# Autodesk Inventor part: Roller Chain
Saved by Autodesk Inventor 2016 (Build 200138000, 138)
## iProperties
Created: 2016-05-10
Part Number: Roller Chain
Material: Generic
Document SubType Name: Modeling
Designer: hesaon
Density: 1 g/cm^3
Appearance: Clear - Blue
CustomPartVersion: 1
Author: hesaon
Autodesk Inventor part; units mm, degrees
ref_plane "Work Plane2" through (-104.6542, 0, 0) normal (-1, 0, 0) x (0, 0, 1)
ref_plane "Work Plane3" through (200, 0, 0) normal (-0.9133742, 0.4071211, 0) x (0, 0, 1)
sketch "Path" plane through (0, 0, 0) normal (0, 0, 1) x (1, 0, 0)
  arc A0 (-103.7053, 31.9399) -> (-103.7053, -31.9399) centre (-104.6542, 0) ccw
  arc A1 (200.6803, -22.8963) -> (200.6803, 22.8963) centre (200, 0) ccw
  line L0 (200.6803, -22.8963) -> (-103.7053, -31.9399)
  line L1 (-103.7053, 31.9399) -> (200.6803, 22.8963)
  dimension "d31" = 8.26
  constraints: 4 end point, 4 point on circle, 2 centre point
ref_plane "Section Plane" through (-103.7053, -31.9399, 0) normal (0.9995589, 0.0296981, 0) x (0, 0, 1)
sketch "Section Sketch" plane through (-103.7053, -31.9399, 0) normal (0.9995589, 0.0296981, 0) x (0, 0, 1)
  line L0 (-6.75, -1.64) -> (6.75, -1.64)
  line L1 (6.75, -1.64) -> (6.75, 1.64)
  line L2 (6.75, 1.64) -> (-6.75, 1.64)
  line L3 (-6.75, 1.64) -> (-6.75, -1.64)
  line L4 (-2.86, -3.175) -> (2.86, -3.175)
  line L5 (2.86, -3.175) -> (2.86, 3.175)
  line L6 (2.86, 3.175) -> (-2.86, 3.175)
  line L7 (-2.86, 3.175) -> (-2.86, -3.175)
  line L8 (-2.86, 0) -> (2.86, 0) construction
  line L9 (-5.16, -4.13) -> (-2.86, -4.13)
  line L10 (-2.86, -4.13) -> (-2.86, 4.13)
  line L11 (-2.86, 4.13) -> (-5.16, 4.13)
  line L12 (-5.16, 4.13) -> (-5.16, -4.13)
  line L13 (2.86, -4.13) -> (5.16, -4.13)
  line L14 (5.16, -4.13) -> (5.16, 4.13)
  line L15 (5.16, 4.13) -> (2.86, 4.13)
  line L16 (2.86, 4.13) -> (2.86, -4.13)
  line L17 (-6.75, 0) -> (6.75, 0) construction
  point P0 (0, 0)
  point P1 (0, 0)
  dimension "d21" = 3.28
  dimension "d22" = 6.35
  dimension "d23" = 5.72
  dimension "d24" = 2.3
  dimension "d31" = 8.26
  dimension "d32" = 13.5
  constraints: 36 end point, 8 midpoint, 8 parallel, 4 horizontal, 4 perpendicular, 3 collinear, 1 coincident, 1 other
  measures "d21" distance between parallel lines of L2 L0
  measures "d22" distance between parallel lines of L6 L4
  measures "d23" distance between parallel lines of L5 L7
  measures "d24" distance between parallel lines of L12 L10
  measures "d31" distance between parallel lines of L11 L9
  measures "d32" distance between parallel lines of L1 L3
sweep "Solid" add profiles "Section Sketch" path "Path"
pattern_of_one "Strand Pattern"
equation "\"d21\" = da_d2"
equation "\"d22\" = da_d1"
equation "\"d23\" = da_b1"
equation "\"d24\" = da_t1 + da_t2"
equation "\"d30\" = da_pt"
equation "\"da_p\" = 9.525"
equation "\"da_b1\" = 5.72"
equation "\"da_h2\" = 8.26"
equation "\"da_h3\" = 8.26"
equation "\"da_d1\" = 6.35"
equation "\"da_d2\" = 3.28"
equation "\"da_pt\" = 10.24"
equation "\"da_b\" = 13.5"
equation "\"da_t1\" = 1.3"
equation "\"da_t2\" = 1"
body "Solid1"
